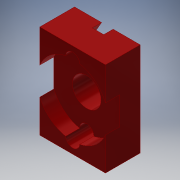
# Autodesk Inventor part: Arm1_BallCasterMount
Saved by Autodesk Inventor 2019 (Build 230136000, 136)
## iProperties
Created: 2021-01-09
Part Number: Arm1_BallCasterMount
Material: Generic
Document SubType Name: Modeling
Designer: Sam
Density: 1 g/cm^3
Appearance: Red
Author: Sam
Autodesk Inventor part; units mm, degrees
ref_plane "YZ Plane" through (0, 0, 0) normal (1, 0, 0) x (0, 1, 0)
ref_plane "XZ Plane" through (0, 0, 0) normal (0, 1, 0) x (-1, 0, 0)
ref_plane "XY Plane" through (0, 0, 0) normal (0, 0, 1) x (1, 0, 0)
sketch "Sketch1" plane through (0, 0, 0) normal (0, 0, 1) x (1, 0, 0)
  line L0 (7, 10) -> (-7, 10)
  line L1 (-7, 10) -> (-7, -10)
  line L2 (-7, -10) -> (7, -10)
  line L3 (7, -10) -> (7, 10)
  circle A0 centre (0, 0) radius 3.05
  point P0 (0, -10)
  point P1 (7, 0)
  dimension "d0" = 20
  dimension "d1" = 14
  dimension "d2" = 6.1
  constraints: 8 end point, 2 midpoint, 2 parallel, 1 centre point, 1 coincident, 1 horizontal, 1 horizontal alignment, 1 perpendicular, 1 vertical alignment
  measures "d0" distance of L2.end L0.start
  measures "d1" distance of L1.end L2.end
  measures "d2" diameter of A0
extrude "Extrusion1" add sketch "Sketch1" along normal blind 4.4
sketch "Sketch2" plane through (0, 0, 4.4) normal (0, 0, 1) x (1, 0, 0)
  circle A0 centre (0, 0) radius 3 construction
  circle A1 centre (0, 0) radius 7.5 construction
  circle A2 centre (0, 0) radius 3.05 construction
  line L0 (7, 10) -> (-7, 10) projected
  line L1 (-7, 10) -> (-7, -10) projected
  line L2 (-7, -10) -> (7, -10) projected
  line L3 (7, -10) -> (7, 10) projected
  circle A3 centre (0, 0) radius 7.6
  line L4 (7, -10) -> (7, 10) projected
  line L5 (7, 2.9597) -> (7, 10)
  line L6 (7, 10) -> (-7, 10) projected
  line L7 (7, 10) -> (-7, 10)
  line L8 (-7, 10) -> (-7, 2.9597)
  line L9 (-7, 10) -> (-7, -10) projected
  line L10 (-7, -2.9597) -> (-7, -10)
  line L11 (-7, -10) -> (7, -10)
  line L12 (7, -2.9597) -> (7, -10)
  dimension "d5" = 15.2
  constraints: 12 end point, 4 point on circle, 4 point on line, 2 collinear, 1 centre point, 1 coincident, 1 horizontal, 1 perpendicular, 1 vertical
  measures "d5" diameter of A3
extrude "Extrusion2" add sketch "Sketch2" along normal blind 3 contours L3 A3 L1 L0 | L3 L2 L1 A3
sketch "Sketch4" plane through (0, 0, 0) normal (0, 0, -1) x (-1, 0, 0)
  circle A0 centre (0, 7.366) radius 1.15 projected
  circle A1 centre (0, -7.366) radius 1.15 projected
  circle A2 centre (0, 7.366) radius 1.5
  circle A3 centre (0, -7.366) radius 1.5
  point P0 (0, 0)
  dimension "d11" = 3
  constraints: 2 centre point, 2 coincident, 1 equal radius
  measures "d11" diameter of A3
extrude "Extrusion4" cut sketch "Sketch4" against normal through all contours A0 | A1 | A2 | A3
sketch "Sketch3" plane through (0, 0, 0) normal (0, 0, -1) x (-1, 0, 0)
  circle A0 centre (0, 7.366) radius 1.15 construction
  circle A1 centre (0, -7.366) radius 1.15 construction
  line L0 (2.754, 7.366) -> (1.377, 4.981)
  line L1 (1.377, 4.981) -> (-1.377, 4.981)
  line L2 (-1.377, 4.981) -> (-2.754, 7.366)
  line L3 (-2.754, 7.366) -> (-1.377, 9.751)
  line L4 (-1.377, 9.751) -> (1.377, 9.751)
  line L5 (1.377, 9.751) -> (2.754, 7.366)
  line L6 (1.377, 9.751) -> (1.2332, 10)
  line L7 (-1.377, 9.751) -> (-1.2332, 10)
  line L8 (1.2332, 10) -> (-1.2332, 10)
  line L9 (-7, 10) -> (7, 10) projected
  point P0 (0, 0)
  dimension "d8" = 4.77
  constraints: 18 end point, 2 collinear, 2 point on line, 1 coincident, 1 horizontal alignment, 13 other
  measures "d8" distance between parallel lines of L1 L4
extrude "Extrusion3" cut sketch "Sketch3" against normal blind 2
sketch "Sketch5" plane through (-1.377, 4.981, 0) normal (0, 1, 0) x (1, 0, 0)
  line L0 (-1.377, 0) -> (-1.377, -2) construction
  line L1 (-1.377, 0) -> (-1.377, -1)
  arc A0 (-1.377, -1) -> (-1.377, 0) centre (-1.7436, -0.5) ccw
  point P0 (1.377, 0)
  point P1 (-1.377, -0.5)
  dimension "d15" = 0.62
  dimension "d16" = 0.3666
  constraints: 2 end point, 2 midpoint, 2 point on circle, 1 centre point, 1 horizontal alignment
  measures "d15" radius of A0
  measures "d16" distance from line of L0 A0.centre
extrude "Extrusion5" add sketch "Sketch5" along normal blind 3
pattern_circular "Circular Pattern1" count 4 over 180 about axis through (0, 7.366, 0) along (0, 0, 1) of "Extrusion5"
mirror "Mirror1" about plane through (0, 0, 0) normal (0, 1, 0) of "Extrusion3", "Extrusion5", "Circular Pattern1"
body "Solid1"
